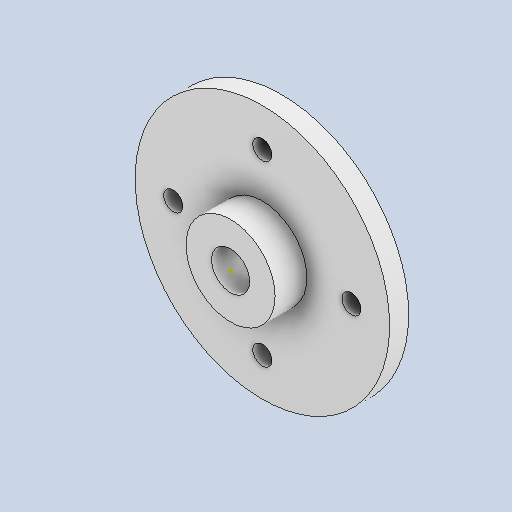
# Autodesk Inventor part: RD010_ギアDS0.5-80
Saved by Autodesk Inventor 2022 (Build 260153000, 153)
## iProperties
Created: 2021-10-14
Part Number: RD010_ギアDS0.5-80
Material: PVC、無可塑
Document SubType Name: Modeling
Designer: gilte
Density: 1.29 g/cm^3
Appearance: 滑らか - 白
Author: gilte
Autodesk Inventor part; units mm, degrees
ref_plane "YZ Plane" through (0, 0, 0) normal (1, 0, 0) x (0, 1, 0)
ref_plane "XZ Plane" through (0, 0, 0) normal (0, 1, 0) x (-1, 0, 0)
ref_plane "XY Plane" through (0, 0, 0) normal (0, 0, 1) x (1, 0, 0)
sketch "スケッチ1" plane through (0, 0, 0) normal (0, 0, 1) x (1, 0, 0)
  circle A0 centre (0, 0) radius 20
  dimension "d0" = 40
  constraints: 1 centre point, 1 coincident
  measures "d0" diameter of A0
extrude "押し出し1" add sketch "スケッチ1" along normal blind 3
sketch "スケッチ2" plane through (0, 0, 3) normal (0, 0, 1) x (1, 0, 0)
  circle A0 centre (0, 0) radius 7
  dimension "d3" = 14
  constraints: 1 centre point, 1 coincident
  measures "d3" diameter of A0
extrude "押し出し2" add sketch "スケッチ2" along normal blind 5
sketch "スケッチ3" plane through (0, 0, 8) normal (0, 0, 1) x (1, 0, 0)
  circle A0 centre (0, 0) radius 3
  dimension "d6" = 6
  constraints: 1 centre point, 1 coincident
  measures "d6" diameter of A0
extrude "押し出し3" cut sketch "スケッチ3" against normal through all
sketch "スケッチ4" plane through (0, 0, 0) normal (0, 0, -1) x (-1, 0, 0)
  point P0 (0, 0)
  point P1 (0, 14)
  point P2 (0, -14)
  point P3 (14, 0)
  point P4 (-14, 0)
  dimension "d9" = 28
  dimension "d10" = 28
  dimension "d11" = 14
  dimension "d12" = 14
  constraints: 2 horizontal alignment, 2 vertical alignment
  measures "d9" distance of point (-14, 0) point (14, 0)
  measures "d10" distance of point (0, 14) point (0, -14)
  measures "d11" distance of point (0, 0) point (14, 0)
  measures "d12" distance of point (0, 14) point (0, 0)
hole "穴1" at (0, 14, 0) at (0, -14, 0) at (-14, 0, 0) at (14, 0, 0) direction (0, 0, 1) diameter 3 end through all
sketch "スケッチ5" plane through (0, 0, 8) normal (0, 0, 1) x (1, 0, 0)
  point P0 (0, 0)
sketch "スケッチ6" plane through (0, 0, 0) normal (1, 0, 0) x (0, 1, 0)
  point P0 (0, 0)
equation "\"d11\" = 0.5 * d9"
equation "\"d12\" = 0.5 * d10"
